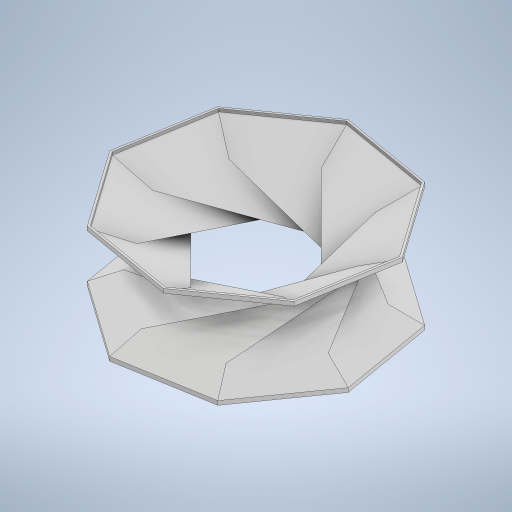
# Autodesk Inventor part: 팔각형 OV-PAM 층 한개
Saved by Autodesk Inventor 2024 (Build 280153000, 153)
## iProperties
Created: 2023-06-16
Part Number: 팔각형 OV-PAM 층 한개
Material: 일반
Document SubType Name: Modeling
Designer: jsw
Density: 1 g/cm^3
Appearance: 기본값
Author: jsw
Autodesk Inventor part; units mm, degrees
sketch "스케치1" plane through (0, 0, 0) normal (0, 1, 0) x (-1, 0, 0)
  line L0 (-35.6097, 14.75) -> (-14.75, 35.6097)
  line L1 (-14.75, 35.6097) -> (14.75, 35.6097)
  line L2 (14.75, 35.6097) -> (35.6097, 14.75)
  line L3 (35.6097, 14.75) -> (35.6097, -14.75)
  line L4 (35.6097, -14.75) -> (14.75, -35.6097)
  line L5 (14.75, -35.6097) -> (-14.75, -35.6097)
  line L6 (-14.75, -35.6097) -> (-35.6097, -14.75)
  line L7 (-35.6097, -14.75) -> (-35.6097, 14.75)
  line L8 (-14.9985, 36.2097) -> (14.9985, 36.2097)
  line L9 (14.9985, 36.2097) -> (36.2097, 14.9985)
  line L10 (36.2097, 14.9985) -> (36.2097, -14.9985)
  line L11 (36.2097, -14.9985) -> (14.9985, -36.2097)
  line L12 (14.9985, -36.2097) -> (-14.9985, -36.2097)
  line L13 (-14.9985, -36.2097) -> (-36.2097, -14.9985)
  line L14 (-36.2097, -14.9985) -> (-36.2097, 14.9985)
  line L15 (-36.2097, 14.9985) -> (-14.9985, 36.2097)
  point P0 (0, 0)
  point P1 (0, 0)
  point P2 (0, 0)
  dimension "d0" = 29.5
  dimension "d2" = 0.6
  constraints: 32 end point, 2 coincident, 2 horizontal, 34 other
  measures "d0" distance of L0.end L1.end
  measures "d2" distance between parallel lines of L10 L3
extrude "돌출2" add sketch "스케치1" along normal blind 24 contours L0 L1 L2 L3 L4 L5 L6 L7 | L8 L9 L10 L11 L12 L13 L14 L15
sketch "스케치33" plane through (14.9985, 0, -36.2097) normal (0, 0, -1) x (-1, 0, 0)
  line L0 (0, 0) -> (0, 24) projected
  line L1 (0, 0) -> (-21.2111, 0) projected
  line L2 (0, 12) -> (-21.2111, 0)
  line L3 (0, 12) -> (21.2111, 24)
  line L4 (29.9971, 24) -> (0, 24) projected
  line L5 (51.2082, 24) -> (29.9971, 24) projected
  line L6 (51.2082, 24) -> (29.9971, 12)
  line L7 (29.9971, 0) -> (29.9971, 24) projected
  line L8 (29.9971, 12) -> (8.7859, 0)
  line L9 (29.9971, 0) -> (0, 0) projected
  line L10 (-21.2111, 0) -> (51.2082, 24)
  point P0 (14.9985, 0)
  constraints: 10 end point, 2 collinear, 2 midpoint, 2 point on line
ref_plane "작업 평면30" through (-6.2126, 24, -36.2097) normal (0.2874189, 0.867278, 0.4064717) x (-0.8164966, 0, 0.5773503)
extrude "돌출27" cut sketch "스케치33" against normal up to surface contours L3 L4 L7 L10 L0 | L0 L10 L2 | L7 L5 L10 surface through (-6.2126, 24, -36.2097) normal (0.2874189, 0.867278, 0.4064717)
sketch "스케치34" plane through (14.9985, 0, -36.2097) normal (0, 0, -1) x (-1, 0, 0)
  line L0 (-21.2111, 0) -> (0, 0) projected
  line L1 (51.2082, 0) -> (51.2082, 24) projected
  line L2 (-21.2111, 0) -> (51.2082, 24)
  line L3 (51.2082, 24) -> (51.2082, 0)
  line L4 (51.2082, 12) -> (29.9971, 12)
  line L5 (29.9971, 0) -> (29.9971, 16.9706) projected
  line L6 (29.9971, 12) -> (51.2082, 24)
  line L7 (29.9971, 12) -> (8.7859, 0)
  line L8 (0, 0) -> (29.9971, 0) projected
  line L9 (8.7859, 0) -> (-21.2111, 0)
  point P0 (14.9985, 0)
  constraints: 12 end point, 2 horizontal, 2 point on line, 1 collinear, 1 midpoint, 1 vertical
ref_plane "작업 평면31" through (36.2097, 0, -14.9985) normal (-0.2874189, -0.867278, 0.4064717) x (-0.9492315, 0.3145785, 0)
extrude "돌출28" cut sketch "스케치34" against normal up to surface contours L2 L5 L7 L8 L0 | L2 L6 L5 surface through (36.2097, 0, -14.9985) normal (-0.2874189, -0.867278, 0.4064717)
pattern_circular "원형 패턴7" count 8 over 360 about axis through (0, -10, 0) along (0, 1, 0) of "돌출28", "돌출27"
ref_plane "작업 평면32" through (0, 12, 0) normal (0, 1, 0) x (1, 0, 0)
sketch "스케치35" plane through (0, 24, 0) normal (0, 1, 0) x (1, 0, 0)
  line L0 (19.1403, 30.3524) -> (-7.9282, 34.9966) projected
  line L1 (-7.9282, 34.9966) -> (-30.3524, 19.1403) projected
  line L2 (-30.3524, 19.1403) -> (-34.9966, -7.9282) projected
  line L3 (-34.9966, -7.9282) -> (-19.1403, -30.3524) projected
  line L4 (-19.1403, -30.3524) -> (7.9282, -34.9966) projected
  line L5 (7.9282, -34.9966) -> (30.3524, -19.1403) projected
  line L6 (30.3524, -19.1403) -> (34.9966, 7.9282) projected
  line L7 (34.9966, 7.9282) -> (19.1403, 30.3524) projected
  point P0 (0, 0)
extrude "돌출29" add sketch "스케치35" along normal blind 1.2
sketch "스케치36" plane through (0, 0, 0) normal (0, -1, 0) x (1, 0, 0)
  line L0 (30.3524, -19.1403) -> (34.9966, 7.9282) projected
  line L1 (34.9966, 7.9282) -> (19.1403, 30.3524) projected
  line L2 (19.1403, 30.3524) -> (-7.9282, 34.9966) projected
  line L3 (-7.9282, 34.9966) -> (-30.3524, 19.1403) projected
  line L4 (-30.3524, 19.1403) -> (-34.9966, -7.9282) projected
  line L5 (-34.9966, -7.9282) -> (-19.1403, -30.3524) projected
  line L6 (-19.1403, -30.3524) -> (7.9282, -34.9966) projected
  line L7 (7.9282, -34.9966) -> (30.3524, -19.1403) projected
  point P0 (0, 0)
extrude "돌출30" add sketch "스케치36" along normal blind 1.2
shell "쉘9" thickness 0.6 removed faces 2 at (-1.0946, 25.2, -4.832) at (2.6427, -1.2, -11.6655)
